Autodesk Inventor part; units mm, degrees
(part 2 of 3)
  line L298 (-57.4722, -60.9676) -> (-57.4397, -60.8956) projected
  line L299 (-57.4397, -60.8956) -> (-57.4038, -60.8255) projected
  line L300 (-57.4038, -60.8255) -> (-57.3646, -60.7575) projected
  line L301 (-57.3646, -60.7575) -> (-57.3224, -60.6916) projected
  line L302 (-57.3224, -60.6916) -> (-57.2771, -60.6279) projected
  line L303 (-57.2771, -60.6279) -> (-57.2288, -60.5665) projected
  line L304 (-57.2288, -60.5665) -> (-57.1777, -60.5075) projected
  line L305 (-57.1777, -60.5075) -> (-57.1239, -60.4511) projected
  line L306 (-57.1239, -60.4511) -> (-57.0675, -60.3973) projected
  line L307 (-57.0675, -60.3973) -> (-57.0085, -60.3462) projected
  line L308 (-57.0085, -60.3462) -> (-56.9471, -60.298) projected
  line L309 (-56.9471, -60.298) -> (-56.8834, -60.2527) projected
  line L310 (-56.8834, -60.2527) -> (-56.8175, -60.2104) projected
  line L311 (-56.8175, -60.2104) -> (-56.7494, -60.1713) projected
  line L312 (-56.7494, -60.1713) -> (-56.6793, -60.1354) projected
  line L313 (-56.6793, -60.1354) -> (-56.6073, -60.1029) projected
  line L314 (-56.6073, -60.1029) -> (-56.5335, -60.0738) projected
  line L315 (-56.5335, -60.0738) -> (-56.458, -60.0483) projected
  line L316 (-56.458, -60.0483) -> (-56.3809, -60.0264) projected
  line L317 (-56.3809, -60.0264) -> (-56.3023, -60.0083) projected
  line L318 (-56.3023, -60.0083) -> (-56.2223, -59.994) projected
  line L319 (-56.2223, -59.994) -> (-56.141, -59.9837) projected
  line L320 (-59.9853, -67.0602) -> (-59.9791, -67.1428) projected
  line L321 (-59.9791, -67.1428) -> (-59.977, -67.2264) projected
  line L322 (-59.977, -67.2264) -> (-59.9792, -67.31) projected
  line L323 (-59.9792, -67.31) -> (-59.9855, -67.3925) projected
  line L324 (-59.9855, -67.3925) -> (-59.9958, -67.4738) projected
  line L325 (-59.9958, -67.4738) -> (-60.0102, -67.5539) projected
  line L326 (-60.0102, -67.5539) -> (-60.0284, -67.6325) projected
  line L327 (-60.0284, -67.6325) -> (-60.0503, -67.7096) projected
  line L328 (-60.0503, -67.7096) -> (-60.0759, -67.7851) projected
  line L329 (-60.0759, -67.7851) -> (-60.105, -67.8588) projected
  line L330 (-60.105, -67.8588) -> (-60.1376, -67.9308) projected
  line L331 (-60.1376, -67.9308) -> (-60.1735, -68.0009) projected
  line L332 (-60.1735, -68.0009) -> (-60.2126, -68.0689) projected
  line L333 (-60.2126, -68.0689) -> (-60.2549, -68.1348) projected
  line L334 (-60.2549, -68.1348) -> (-60.3003, -68.1985) projected
  line L335 (-60.3003, -68.1985) -> (-60.3486, -68.2599) projected
  line L336 (-60.3486, -68.2599) -> (-60.3997, -68.3188) projected
  line L337 (-60.3997, -68.3188) -> (-60.4535, -68.3752) projected
  line L338 (-60.4535, -68.3752) -> (-60.5099, -68.429) projected
  line L339 (-60.5099, -68.429) -> (-60.5689, -68.48) projected
  line L340 (-60.5689, -68.48) -> (-60.6303, -68.5283) projected
  line L341 (-60.6303, -68.5283) -> (-60.6941, -68.5735) projected
  line L342 (-60.6941, -68.5735) -> (-60.76, -68.6158) projected
  line L343 (-60.76, -68.6158) -> (-60.8281, -68.6549) projected
  line L344 (-60.8281, -68.6549) -> (-60.8982, -68.6907) projected
  line L345 (-60.8982, -68.6907) -> (-60.9702, -68.7232) projected
  line L346 (-60.9702, -68.7232) -> (-61.044, -68.7523) projected
  line L347 (-61.044, -68.7523) -> (-61.1195, -68.7778) projected
  line L348 (-61.1195, -68.7778) -> (-61.1966, -68.7997) projected
  line L349 (-61.1966, -68.7997) -> (-61.2752, -68.8178) projected
  line L350 (-61.2752, -68.8178) -> (-61.3553, -68.832) projected
  line L351 (-61.3553, -68.832) -> (-61.4366, -68.8423) projected
  line L352 (-61.4366, -68.8423) -> (-61.5191, -68.8486) projected
  line L353 (-61.5191, -68.8486) -> (-61.6028, -68.8506) projected
  line L354 (-61.6028, -68.8506) -> (-61.6864, -68.8485) projected
  line L355 (-61.6864, -68.8485) -> (-61.7689, -68.8422) projected
  line L356 (-61.7689, -68.8422) -> (-61.8502, -68.8318) projected
  line L357 (-61.8502, -68.8318) -> (-61.9302, -68.8175) projected
  line L358 (-61.9302, -68.8175) -> (-62.0088, -68.7993) projected
  line L359 (-62.0088, -68.7993) -> (-62.0859, -68.7774) projected
  line L360 (-62.0859, -68.7774) -> (-62.1614, -68.7518) projected
  line L361 (-62.1614, -68.7518) -> (-62.2352, -68.7226) projected
  line L362 (-62.2352, -68.7226) -> (-62.3072, -68.6901) projected
  line L363 (-62.3072, -68.6901) -> (-62.3772, -68.6542) projected
  line L364 (-62.3772, -68.6542) -> (-62.4453, -68.615) projected
  line L365 (-62.4453, -68.615) -> (-62.5112, -68.5727) projected
  line L366 (-62.5112, -68.5727) -> (-62.5749, -68.5274) projected
  line L367 (-62.5749, -68.5274) -> (-62.6362, -68.4791) projected
  line L368 (-62.6362, -68.4791) -> (-62.6952, -68.428) projected
  line L369 (-62.6952, -68.428) -> (-62.7516, -68.3742) projected
  line L370 (-62.7516, -68.3742) -> (-62.8054, -68.3177) projected
  line L371 (-62.8054, -68.3177) -> (-62.8564, -68.2587) projected
  line L372 (-62.8564, -68.2587) -> (-62.9046, -68.1973) projected
  line L373 (-62.9046, -68.1973) -> (-62.9499, -68.1336) projected
  line L374 (-62.9499, -68.1336) -> (-62.9921, -68.0676) projected
  line L375 (-62.9921, -68.0676) -> (-63.0312, -67.9996) projected
  line L376 (-63.0312, -67.9996) -> (-63.0671, -67.9295) projected
  line L377 (-63.0671, -67.9295) -> (-63.0996, -67.8575) projected
  line L378 (-63.0996, -67.8575) -> (-63.1287, -67.7837) projected
  line L379 (-63.1287, -67.7837) -> (-63.1542, -67.7082) projected
  line L380 (-63.1542, -67.7082) -> (-63.176, -67.631) projected
  line L381 (-63.176, -67.631) -> (-63.1941, -67.5524) projected
  line L382 (-63.1941, -67.5524) -> (-63.2084, -67.4724) projected
  line L383 (-63.2084, -67.4724) -> (-63.2187, -67.391) projected
  line L384 (-63.2187, -67.391) -> (-63.2249, -67.3085) projected
  line L385 (-63.2249, -67.3085) -> (-63.227, -67.2249) projected
  line L386 (-63.227, -67.2249) -> (-63.2249, -67.1413) projected
  line L387 (-63.2249, -67.1413) -> (-63.2185, -67.0588) projected
  line L388 (-63.2185, -67.0588) -> (-63.2082, -66.9774) projected
  line L389 (-63.2082, -66.9774) -> (-63.1938, -66.8974) projected
  line L390 (-63.1938, -66.8974) -> (-63.1757, -66.8188) projected
  line L391 (-63.1757, -66.8188) -> (-63.1537, -66.7417) projected
  line L392 (-63.1537, -66.7417) -> (-63.1281, -66.6662) projected
  line L393 (-63.1281, -66.6662) -> (-63.099, -66.5924) projected
  line L394 (-63.099, -66.5924) -> (-63.0664, -66.5205) projected
  line L395 (-63.0664, -66.5205) -> (-63.0305, -66.4504) projected
  line L396 (-63.0305, -66.4504) -> (-62.9914, -66.3824) projected
  line L397 (-62.9914, -66.3824) -> (-62.9491, -66.3165) projected
  line L398 (-62.9491, -66.3165) -> (-62.9037, -66.2528) projected
  line L399 (-62.9037, -66.2528) -> (-62.8555, -66.1914) projected
  line L400 (-62.8555, -66.1914) -> (-62.8044, -66.1325) projected
  line L401 (-62.8044, -66.1325) -> (-62.7505, -66.0761) projected
  line L402 (-62.7505, -66.0761) -> (-62.6941, -66.0223) projected
  line L403 (-62.6941, -66.0223) -> (-62.6351, -65.9712) projected
  line L404 (-62.6351, -65.9712) -> (-62.5737, -65.923) projected
  line L405 (-62.5737, -65.923) -> (-62.5099, -65.8777) projected
  line L406 (-62.5099, -65.8777) -> (-62.444, -65.8355) projected
  line L407 (-62.444, -65.8355) -> (-62.3759, -65.7964) projected
  line L408 (-62.3759, -65.7964) -> (-62.3058, -65.7606) projected
  line L409 (-62.3058, -65.7606) -> (-62.2338, -65.7281) projected
  line L410 (-62.2338, -65.7281) -> (-62.16, -65.699) projected
  line L411 (-62.16, -65.699) -> (-62.0845, -65.6735) projected
  line L412 (-62.0845, -65.6735) -> (-62.0074, -65.6516) projected
  line L413 (-62.0074, -65.6516) -> (-61.9288, -65.6335) projected
  line L414 (-61.9288, -65.6335) -> (-61.8487, -65.6193) projected
  line L415 (-61.8487, -65.6193) -> (-61.7674, -65.609) projected
  line L416 (-61.7674, -65.609) -> (-61.6849, -65.6027) projected
  line L417 (-61.6849, -65.6027) -> (-61.6013, -65.6006) projected
  line L418 (-61.6013, -65.6006) -> (-61.5176, -65.6028) projected
  line L419 (-61.5176, -65.6028) -> (-61.4351, -65.6091) projected
  line L420 (-61.4351, -65.6091) -> (-61.3538, -65.6195) projected
  line L421 (-61.3538, -65.6195) -> (-61.2738, -65.6338) projected
  line L422 (-61.2738, -65.6338) -> (-61.1952, -65.652) projected
  line L423 (-61.1952, -65.652) -> (-61.1181, -65.6739) projected
  line L424 (-61.1181, -65.6739) -> (-61.0426, -65.6995) projected
  line L425 (-61.0426, -65.6995) -> (-60.9688, -65.7286) projected
  line L426 (-60.9688, -65.7286) -> (-60.8968, -65.7612) projected
  line L427 (-60.8968, -65.7612) -> (-60.8268, -65.7971) projected
  line L428 (-60.8268, -65.7971) -> (-60.7587, -65.8363) projected
  line L429 (-60.7587, -65.8363) -> (-60.6928, -65.8786) projected
  line L430 (-60.6928, -65.8786) -> (-60.6291, -65.9239) projected
  line L431 (-60.6291, -65.9239) -> (-60.5678, -65.9722) projected
  line L432 (-60.5678, -65.9722) -> (-60.5088, -66.0233) projected
  line L433 (-60.5088, -66.0233) -> (-60.4524, -66.0771) projected
  line L434 (-60.4524, -66.0771) -> (-60.3987, -66.1336) projected
  line L435 (-60.3987, -66.1336) -> (-60.3476, -66.1926) projected
  line L436 (-60.3476, -66.1926) -> (-60.2994, -66.254) projected
  line L437 (-60.2994, -66.254) -> (-60.2541, -66.3177) projected
  line L438 (-60.2541, -66.3177) -> (-60.2119, -66.3837) projected
  line L439 (-60.2119, -66.3837) -> (-60.1728, -66.4517) projected
  line L440 (-60.1728, -66.4517) -> (-60.1369, -66.5218) projected
  line L441 (-60.1369, -66.5218) -> (-60.1044, -66.5938) projected
  line L442 (-60.1044, -66.5938) -> (-60.0754, -66.6676) projected
  line L443 (-60.0754, -66.6676) -> (-60.0498, -66.7431) projected
  line L444 (-60.0498, -66.7431) -> (-60.028, -66.8202) projected
  line L445 (-60.028, -66.8202) -> (-60.0099, -66.8989) projected
  line L446 (-60.0099, -66.8989) -> (-59.9956, -66.9789) projected
  line L447 (-59.9956, -66.9789) -> (-59.9853, -67.0602) projected
  line L448 (-63.2161, -56.1402) -> (-63.2223, -56.0577) projected
  line L449 (-63.2223, -56.0577) -> (-63.2244, -55.9741) projected
  line L450 (-63.2244, -55.9741) -> (-63.2223, -55.8904) projected
  line L451 (-63.2223, -55.8904) -> (-63.216, -55.8079) projected
  line L452 (-63.216, -55.8079) -> (-63.2056, -55.7266) projected
  line L453 (-63.2056, -55.7266) -> (-63.1913, -55.6466) projected
  line L454 (-63.1913, -55.6466) -> (-63.1732, -55.568) projected
  line L455 (-63.1732, -55.568) -> (-63.1512, -55.4909) projected
  line L456 (-63.1512, -55.4909) -> (-63.1257, -55.4154) projected
  line L457 (-63.1257, -55.4154) -> (-63.0966, -55.3416) projected
  line L458 (-63.0966, -55.3416) -> (-63.064, -55.2696) projected
  line L459 (-63.064, -55.2696) -> (-63.0281, -55.1995) projected
  line L460 (-63.0281, -55.1995) -> (-62.9889, -55.1315) projected
  line L461 (-62.9889, -55.1315) -> (-62.9467, -55.0656) projected
  line L462 (-62.9467, -55.0656) -> (-62.9013, -55.0019) projected
  line L463 (-62.9013, -55.0019) -> (-62.8531, -54.9405) projected
  line L464 (-62.8531, -54.9405) -> (-62.802, -54.8816) projected
  line L465 (-62.802, -54.8816) -> (-62.7482, -54.8251) projected
  line L466 (-62.7482, -54.8251) -> (-62.6917, -54.7714) projected
  line L467 (-62.6917, -54.7714) -> (-62.6327, -54.7203) projected
  line L468 (-62.6327, -54.7203) -> (-62.5713, -54.6721) projected
  line L469 (-62.5713, -54.6721) -> (-62.5076, -54.6268) projected
  line L470 (-62.5076, -54.6268) -> (-62.4417, -54.5845) projected
  line L471 (-62.4417, -54.5845) -> (-62.3736, -54.5454) projected
  line L472 (-62.3736, -54.5454) -> (-62.3035, -54.5096) projected
  line L473 (-62.3035, -54.5096) -> (-62.2315, -54.477) projected
  line L474 (-62.2315, -54.477) -> (-62.1577, -54.448) projected
  line L475 (-62.1577, -54.448) -> (-62.0822, -54.4224) projected
  line L476 (-62.0822, -54.4224) -> (-62.0051, -54.4006) projected
  line L477 (-62.0051, -54.4006) -> (-61.9265, -54.3824) projected
  line L478 (-61.9265, -54.3824) -> (-61.8465, -54.3682) projected
  line L479 (-61.8465, -54.3682) -> (-61.7651, -54.3579) projected
  line L480 (-61.7651, -54.3579) -> (-61.6826, -54.3516) projected
  line L481 (-61.6826, -54.3516) -> (-61.599, -54.3495) projected
  line L482 (-61.599, -54.3495) -> (-61.5154, -54.3517) projected
  line L483 (-61.5154, -54.3517) -> (-61.4328, -54.358) projected
  line L484 (-61.4328, -54.358) -> (-61.3515, -54.3683) projected
  line L485 (-61.3515, -54.3683) -> (-61.2715, -54.3826) projected
  line L486 (-61.2715, -54.3826) -> (-61.1929, -54.4008) projected
  line L487 (-61.1929, -54.4008) -> (-61.1158, -54.4227) projected
  line L488 (-61.1158, -54.4227) -> (-61.0403, -54.4483) projected
  line L489 (-61.0403, -54.4483) -> (-60.9665, -54.4774) projected
  line L490 (-60.9665, -54.4774) -> (-60.8945, -54.51) projected
  line L491 (-60.8945, -54.51) -> (-60.8245, -54.5459) projected
  line L492 (-60.8245, -54.5459) -> (-60.7564, -54.585) projected
  line L493 (-60.7564, -54.585) -> (-60.6905, -54.6273) projected
  line L494 (-60.6905, -54.6273) -> (-60.6268, -54.6726) projected
  line L495 (-60.6268, -54.6726) -> (-60.5654, -54.7209) projected
  line L496 (-60.5654, -54.7209) -> (-60.5065, -54.772) projected
  line L497 (-60.5065, -54.772) -> (-60.4501, -54.8258) projected
  line L498 (-60.4501, -54.8258) -> (-60.3963, -54.8822) projected
  line L499 (-60.3963, -54.8822) -> (-60.3452, -54.9412) projected
  line L500 (-60.3452, -54.9412) -> (-60.297, -55.0026) projected
  line L501 (-60.297, -55.0026) -> (-60.2517, -55.0663) projected
  line L502 (-60.2517, -55.0663) -> (-60.2095, -55.1323) projected
  line L503 (-60.2095, -55.1323) -> (-60.1703, -55.2003) projected
  line L504 (-60.1703, -55.2003) -> (-60.1345, -55.2704) projected
  line L505 (-60.1345, -55.2704) -> (-60.102, -55.3424) projected
  line L506 (-60.102, -55.3424) -> (-60.0729, -55.4162) projected
  line L507 (-60.0729, -55.4162) -> (-60.0474, -55.4917) projected
  line L508 (-60.0474, -55.4917) -> (-60.0255, -55.5688) projected
  line L509 (-60.0255, -55.5688) -> (-60.0074, -55.6475) projected
  line L510 (-60.0074, -55.6475) -> (-59.9931, -55.7275) projected
  line L511 (-59.9931, -55.7275) -> (-59.9828, -55.8088) projected
  line L512 (-59.9828, -55.8088) -> (-59.9765, -55.8914) projected
  line L513 (-59.9765, -55.8914) -> (-59.9744, -55.975) projected
  line L514 (-59.9744, -55.975) -> (-59.9766, -56.0586) projected
  line L515 (-59.9766, -56.0586) -> (-59.9829, -56.1411) projected
  line L516 (-59.9829, -56.1411) -> (-59.9932, -56.2224) projected
  line L517 (-59.9932, -56.2224) -> (-60.0075, -56.3025) projected
  line L518 (-60.0075, -56.3025) -> (-60.0257, -56.3811) projected
  line L519 (-60.0257, -56.3811) -> (-60.0476, -56.4582) projected
  line L520 (-60.0476, -56.4582) -> (-60.0732, -56.5337) projected
  line L521 (-60.0732, -56.5337) -> (-60.1023, -56.6075) projected
  line L522 (-60.1023, -56.6075) -> (-60.1349, -56.6794) projected
  line L523 (-60.1349, -56.6794) -> (-60.1708, -56.7495) projected
  line L524 (-60.1708, -56.7495) -> (-60.2099, -56.8175) projected
  line L525 (-60.2099, -56.8175) -> (-60.2522, -56.8834) projected
  line L526 (-60.2522, -56.8834) -> (-60.2975, -56.9471) projected
  line L527 (-60.2975, -56.9471) -> (-60.3458, -57.0085) projected
  line L528 (-60.3458, -57.0085) -> (-60.3969, -57.0675) projected
  line L529 (-60.3969, -57.0675) -> (-60.4507, -57.1239) projected
  line L530 (-60.4507, -57.1239) -> (-60.5072, -57.1777) projected
  line L531 (-60.5072, -57.1777) -> (-60.5661, -57.2287) projected
  line L532 (-60.5661, -57.2287) -> (-60.6275, -57.277) projected
  line L533 (-60.6275, -57.277) -> (-60.6913, -57.3222) projected
  line L534 (-60.6913, -57.3222) -> (-60.7572, -57.3645) projected
  line L535 (-60.7572, -57.3645) -> (-60.8253, -57.4036) projected
  line L536 (-60.8253, -57.4036) -> (-60.8953, -57.4395) projected
  line L537 (-60.8953, -57.4395) -> (-60.9673, -57.472) projected
  line L538 (-60.9673, -57.472) -> (-61.0411, -57.5011) projected
  line L539 (-61.0411, -57.5011) -> (-61.1166, -57.5266) projected
  line L540 (-61.1166, -57.5266) -> (-61.1938, -57.5485) projected
  line L541 (-61.1938, -57.5485) -> (-61.2724, -57.5666) projected
  line L542 (-61.2724, -57.5666) -> (-61.3524, -57.5809) projected
  line L543 (-61.3524, -57.5809) -> (-61.4337, -57.5912) projected
  line L544 (-61.4337, -57.5912) -> (-61.5163, -57.5974) projected
  line L545 (-61.5163, -57.5974) -> (-61.5999, -57.5995) projected
  line L546 (-61.5999, -57.5995) -> (-61.6835, -57.5974) projected
  line L547 (-61.6835, -57.5974) -> (-61.766, -57.5911) projected
  line L548 (-61.766, -57.5911) -> (-61.8474, -57.5807) projected
  line L549 (-61.8474, -57.5807) -> (-61.9274, -57.5664) projected
  line L550 (-61.9274, -57.5664) -> (-62.006, -57.5482) projected
  line L551 (-62.006, -57.5482) -> (-62.0831, -57.5263) projected
  line L552 (-62.0831, -57.5263) -> (-62.1586, -57.5008) projected
  line L553 (-62.1586, -57.5008) -> (-62.2324, -57.4716) projected
  line L554 (-62.2324, -57.4716) -> (-62.3044, -57.4391) projected
  line L555 (-62.3044, -57.4391) -> (-62.3744, -57.4032) projected
  line L556 (-62.3744, -57.4032) -> (-62.4424, -57.364) projected
  line L557 (-62.4424, -57.364) -> (-62.5084, -57.3217) projected
  line L558 (-62.5084, -57.3217) -> (-62.5721, -57.2764) projected
  line L559 (-62.5721, -57.2764) -> (-62.6334, -57.2282) projected
  line L560 (-62.6334, -57.2282) -> (-62.6924, -57.1771) projected
  line L561 (-62.6924, -57.1771) -> (-62.7488, -57.1232) projected
  line L562 (-62.7488, -57.1232) -> (-62.8026, -57.0668) projected
  line L563 (-62.8026, -57.0668) -> (-62.8537, -57.0078) projected
  line L564 (-62.8537, -57.0078) -> (-62.9019, -56.9464) projected
  line L565 (-62.9019, -56.9464) -> (-62.9472, -56.8827) projected
  line L566 (-62.9472, -56.8827) -> (-62.9894, -56.8167) projected
  line L567 (-62.9894, -56.8167) -> (-63.0285, -56.7487) projected
  line L568 (-63.0285, -56.7487) -> (-63.0644, -56.6786) projected
  line L569 (-63.0644, -56.6786) -> (-63.0969, -56.6066) projected
  line L570 (-63.0969, -56.6066) -> (-63.126, -56.5328) projected
  line L571 (-63.126, -56.5328) -> (-63.1515, -56.4573) projected
  line L572 (-63.1515, -56.4573) -> (-63.1734, -56.3802) projected
  line L573 (-63.1734, -56.3802) -> (-63.1915, -56.3016) projected
  line L574 (-63.1915, -56.3016) -> (-63.2058, -56.2215) projected
  line L575 (-63.2058, -56.2215) -> (-63.2161, -56.1402) projected
  arc A0 (-52.9038, -71.2653) -> (-48.6, -61.6029) centre (-61.5843, -61.6091) ccw projected
  arc A1 (-48.6, -61.6029) -> (-48.8055, -59.2842) centre (-61.5557, -61.583) ccw projected
  arc A2 (-48.8055, -59.2842) -> (-59.1805, -48.8249) centre (-61.5989, -61.5991) ccw projected
  arc A3 (-59.1805, -48.8249) -> (-74.163, -58.2471) centre (-61.5986, -61.6031) ccw projected
  arc A4 (-74.163, -58.2471) -> (-72.8082, -68.1903) centre (-61.5989, -61.5991) ccw projected
  arc A5 (-72.8082, -68.1903) -> (-52.9038, -71.2653) centre (-61.6004, -61.5999) ccw projected
  point P0 (0, 0)
ref_plane "Work Plane1" through (0, 0, 0) normal (0, 0, 1) x (1, 0, 0)
sketch "Sketch5" plane through (0, 0, 0) normal (0, 0, 1) x (1, 0, 0)
  line L0 (67.06, -63.215) -> (67.1425, -63.2212) projected
  line L1 (67.1425, -63.2212) -> (67.2261, -63.2233) projected
  line L2 (67.2261, -63.2233) -> (67.3097, -63.2211) projected
  line L3 (67.3097, -63.2211) -> (67.3923, -63.2148) projected
  line L4 (67.3923, -63.2148) -> (67.4736, -63.2045) projected
  line L5 (67.4736, -63.2045) -> (67.5536, -63.1902) projected
  line L6 (67.5536, -63.1902) -> (67.6322, -63.172) projected
  line L7 (67.6322, -63.172) -> (67.7093, -63.15) projected
  line L8 (67.7093, -63.15) -> (67.7848, -63.1245) projected
  line L9 (67.7848, -63.1245) -> (67.8586, -63.0953) projected
  line L10 (67.8586, -63.0953) -> (67.9306, -63.0628) projected
  line L11 (67.9306, -63.0628) -> (68.0006, -63.0269) projected
  line L12 (68.0006, -63.0269) -> (68.0686, -62.9877) projected
  line L13 (68.0686, -62.9877) -> (68.1346, -62.9454) projected
  line L14 (68.1346, -62.9454) -> (68.1982, -62.9001) projected
  line L15 (68.1982, -62.9001) -> (68.2596, -62.8518) projected
  line L16 (68.2596, -62.8518) -> (68.3186, -62.8007) projected
  line L17 (68.3186, -62.8007) -> (68.375, -62.7469) projected
  line L18 (68.375, -62.7469) -> (68.4288, -62.6904) projected
  line L19 (68.4288, -62.6904) -> (68.4798, -62.6314) projected
  line L20 (68.4798, -62.6314) -> (68.528, -62.57) projected
  line L21 (68.528, -62.57) -> (68.5733, -62.5063) projected
  line L22 (68.5733, -62.5063) -> (68.6155, -62.4404) projected
  line L23 (68.6155, -62.4404) -> (68.6546, -62.3723) projected
  line L24 (68.6546, -62.3723) -> (68.6905, -62.3022) projected
  line L25 (68.6905, -62.3022) -> (68.723, -62.2302) projected
  line L26 (68.723, -62.2302) -> (68.7521, -62.1564) projected
  line L27 (68.7521, -62.1564) -> (68.7776, -62.0809) projected
  line L28 (68.7776, -62.0809) -> (68.7995, -62.0038) projected
  line L29 (68.7995, -62.0038) -> (68.8176, -61.9252) projected
  line L30 (68.8176, -61.9252) -> (68.8318, -61.8451) projected
  line L31 (68.8318, -61.8451) -> (68.8421, -61.7638) projected
  line L32 (68.8421, -61.7638) -> (68.8484, -61.6813) projected
  line L33 (68.8484, -61.6813) -> (68.8505, -61.5976) projected
  line L34 (68.8505, -61.5976) -> (68.8483, -61.514) projected
  line L35 (68.8483, -61.514) -> (68.842, -61.4315) projected
  line L36 (68.842, -61.4315) -> (68.8316, -61.3502) projected
  line L37 (68.8316, -61.3502) -> (68.8173, -61.2702) projected
  line L38 (68.8173, -61.2702) -> (68.7991, -61.1916) projected
  line L39 (68.7991, -61.1916) -> (68.7772, -61.1144) projected
  line L40 (68.7772, -61.1144) -> (68.7516, -61.039) projected
  line L41 (68.7516, -61.039) -> (68.7225, -60.9652) projected
  line L42 (68.7225, -60.9652) -> (68.6899, -60.8932) projected
  line L43 (68.6899, -60.8932) -> (68.654, -60.8232) projected
  line L44 (68.654, -60.8232) -> (68.6149, -60.7551) projected
  line L45 (68.6149, -60.7551) -> (68.5726, -60.6892) projected
  line L46 (68.5726, -60.6892) -> (68.5272, -60.6255) projected
  line L47 (68.5272, -60.6255) -> (68.479, -60.5641) projected
  line L48 (68.479, -60.5641) -> (68.4279, -60.5052) projected
  line L49 (68.4279, -60.5052) -> (68.374, -60.4488) projected
  line L50 (68.374, -60.4488) -> (68.3176, -60.395) projected
  line L51 (68.3176, -60.395) -> (68.2586, -60.344) projected
  line L52 (68.2586, -60.344) -> (68.1972, -60.2957) projected
  line L53 (68.1972, -60.2957) -> (68.1335, -60.2505) projected
  line L54 (68.1335, -60.2505) -> (68.0675, -60.2082) projected
  line L55 (68.0675, -60.2082) -> (67.9995, -60.1691) projected
  line L56 (67.9995, -60.1691) -> (67.9294, -60.1333) projected
  line L57 (67.9294, -60.1333) -> (67.8574, -60.1007) projected
  line L58 (67.8574, -60.1007) -> (67.7836, -60.0717) projected
  line L59 (67.7836, -60.0717) -> (67.7081, -60.0462) projected
  line L60 (67.7081, -60.0462) -> (67.6309, -60.0243) projected
  line L61 (67.6309, -60.0243) -> (67.5523, -60.0062) projected
  line L62 (67.5523, -60.0062) -> (67.4723, -59.9919) projected
  line L63 (67.4723, -59.9919) -> (67.391, -59.9816) projected
  line L64 (67.391, -59.9816) -> (67.3084, -59.9754) projected
  line L65 (67.3084, -59.9754) -> (67.2248, -59.9733) projected
  line L66 (67.2248, -59.9733) -> (67.1412, -59.9754) projected
  line L67 (67.1412, -59.9754) -> (67.0587, -59.9818) projected
  line L68 (67.0587, -59.9818) -> (66.9773, -59.9921) projected
  line L69 (66.9773, -59.9921) -> (66.8973, -60.0064) projected
  line L70 (66.8973, -60.0064) -> (66.8187, -60.0246) projected
  line L71 (66.8187, -60.0246) -> (66.7416, -60.0465) projected
  line L72 (66.7416, -60.0465) -> (66.6661, -60.0721) projected
  line L73 (66.6661, -60.0721) -> (66.5923, -60.1013) projected
  line L74 (66.5923, -60.1013) -> (66.5204, -60.1338) projected
  line L75 (66.5204, -60.1338) -> (66.4503, -60.1697) projected
  line L76 (66.4503, -60.1697) -> (66.3823, -60.2089) projected
  line L77 (66.3823, -60.2089) -> (66.3164, -60.2512) projected
  line L78 (66.3164, -60.2512) -> (66.2527, -60.2965) projected
  line L79 (66.2527, -60.2965) -> (66.1913, -60.3448) projected
  line L80 (66.1913, -60.3448) -> (66.1324, -60.3959) projected
  line L81 (66.1324, -60.3959) -> (66.0759, -60.4497) projected
  line L82 (66.0759, -60.4497) -> (66.0222, -60.5062) projected
  line L83 (66.0222, -60.5062) -> (65.9711, -60.5652) projected
  line L84 (65.9711, -60.5652) -> (65.9229, -60.6266) projected
  line L85 (65.9229, -60.6266) -> (65.8776, -60.6903) projected
  line L86 (65.8776, -60.6903) -> (65.8354, -60.7562) projected
  line L87 (65.8354, -60.7562) -> (65.7963, -60.8243) projected
  line L88 (65.7963, -60.8243) -> (65.7604, -60.8944) projected
  line L89 (65.7604, -60.8944) -> (65.7279, -60.9664) projected
  line L90 (65.7279, -60.9664) -> (65.6988, -61.0402) projected
  line L91 (65.6988, -61.0402) -> (65.6733, -61.1157) projected
  line L92 (65.6733, -61.1157) -> (65.6515, -61.1928) projected
  line L93 (65.6515, -61.1928) -> (65.6333, -61.2714) projected
  line L94 (65.6333, -61.2714) -> (65.6191, -61.3515) projected
  line L95 (65.6191, -61.3515) -> (65.6088, -61.4328) projected
  line L96 (65.6088, -61.4328) -> (65.6025, -61.5153) projected
  line L97 (65.6025, -61.5153) -> (65.6005, -61.599) projected
  line L98 (65.6005, -61.599) -> (65.6026, -61.6826) projected
  line L99 (65.6026, -61.6826) -> (65.6089, -61.7651) projected
  line L100 (65.6089, -61.7651) -> (65.6193, -61.8464) projected
  line L101 (65.6193, -61.8464) -> (65.6336, -61.9264) projected
  line L102 (65.6336, -61.9264) -> (65.6518, -62.005) projected
  line L103 (65.6518, -62.005) -> (65.6737, -62.0821) projected
  line L104 (65.6737, -62.0821) -> (65.6993, -62.1576) projected
  line L105 (65.6993, -62.1576) -> (65.7284, -62.2314) projected
  line L106 (65.7284, -62.2314) -> (65.761, -62.3034) projected
  line L107 (65.761, -62.3034) -> (65.7969, -62.3734) projected
  line L108 (65.7969, -62.3734) -> (65.8361, -62.4415) projected
  line L109 (65.8361, -62.4415) -> (65.8783, -62.5074) projected
  line L110 (65.8783, -62.5074) -> (65.9237, -62.5711) projected
  line L111 (65.9237, -62.5711) -> (65.9719, -62.6325) projected
  line L112 (65.9719, -62.6325) -> (66.023, -62.6914) projected
  line L113 (66.023, -62.6914) -> (66.0769, -62.7478) projected
  line L114 (66.0769, -62.7478) -> (66.1333, -62.8016) projected
  line L115 (66.1333, -62.8016) -> (66.1923, -62.8526) projected
  line L116 (66.1923, -62.8526) -> (66.2537, -62.9009) projected
  line L117 (66.2537, -62.9009) -> (66.3174, -62.9461) projected
  line L118 (66.3174, -62.9461) -> (66.3834, -62.9884) projected
  line L119 (66.3834, -62.9884) -> (66.4515, -63.0275) projected
  line L120 (66.4515, -63.0275) -> (66.5215, -63.0633) projected
  line L121 (66.5215, -63.0633) -> (66.5935, -63.0959) projected
  line L122 (66.5935, -63.0959) -> (66.6673, -63.1249) projected
  line L123 (66.6673, -63.1249) -> (66.7429, -63.1504) projected
  line L124 (66.7429, -63.1504) -> (66.82, -63.1723) projected
  line L125 (66.82, -63.1723) -> (66.8986, -63.1904) projected
  line L126 (66.8986, -63.1904) -> (66.9786, -63.2047) projected
  line L127 (66.9786, -63.2047) -> (67.06, -63.215) projected
  line L128 (56.141, -59.9837) -> (56.0584, -59.9774) projected
  line L129 (56.0584, -59.9774) -> (55.9748, -59.9753) projected
  line L130 (55.9748, -59.9753) -> (55.8912, -59.9774) projected
  line L131 (55.8912, -59.9774) -> (55.8087, -59.9837) projected
  line L132 (55.8087, -59.9837) -> (55.7273, -59.994) projected
  line L133 (55.7273, -59.994) -> (55.6473, -60.0083) projected
  line L134 (55.6473, -60.0083) -> (55.5687, -60.0265) projected
  line L135 (55.5687, -60.0265) -> (55.4916, -60.0484) projected
  line L136 (55.4916, -60.0484) -> (55.4161, -60.074) projected
  line L137 (55.4161, -60.074) -> (55.3423, -60.1031) projected
  line L138 (55.3423, -60.1031) -> (55.2703, -60.1356) projected
  line L139 (55.2703, -60.1356) -> (55.2003, -60.1715) projected
  line L140 (55.2003, -60.1715) -> (55.1322, -60.2106) projected
  line L141 (55.1322, -60.2106) -> (55.0663, -60.2529) projected
  line L142 (55.0663, -60.2529) -> (55.0026, -60.2982) projected
  line L143 (55.0026, -60.2982) -> (54.9412, -60.3465) projected
  line L144 (54.9412, -60.3465) -> (54.8822, -60.3976) projected
  line L145 (54.8822, -60.3976) -> (54.8258, -60.4514) projected
  line L146 (54.8258, -60.4514) -> (54.772, -60.5078) projected
  line L147 (54.772, -60.5078) -> (54.7209, -60.5668) projected
  line L148 (54.7209, -60.5668) -> (54.6727, -60.6282) projected
  line L149 (54.6727, -60.6282) -> (54.6274, -60.6919) projected
  line L150 (54.6274, -60.6919) -> (54.5852, -60.7578) projected
  line L151 (54.5852, -60.7578) -> (54.546, -60.8259) projected
  line L152 (54.546, -60.8259) -> (54.5102, -60.8959) projected
  line L153 (54.5102, -60.8959) -> (54.4776, -60.9679) projected
  line L154 (54.4776, -60.9679) -> (54.4485, -61.0417) projected
  line L155 (54.4485, -61.0417) -> (54.423, -61.1172) projected
  line L156 (54.423, -61.1172) -> (54.4011, -61.1944) projected
  line L157 (54.4011, -61.1944) -> (54.383, -61.273) projected
  line L158 (54.383, -61.273) -> (54.3687, -61.353) projected
  line L159 (54.3687, -61.353) -> (54.3584, -61.4343) projected
  line L160 (54.3584, -61.4343) -> (54.3521, -61.5169) projected
  line L161 (54.3521, -61.5169) -> (54.35, -61.6005) projected
  line L162 (54.35, -61.6005) -> (54.3521, -61.6841) projected
  line L163 (54.3521, -61.6841) -> (54.3584, -61.7666) projected
  line L164 (54.3584, -61.7666) -> (54.3688, -61.8479) projected
  line L165 (54.3688, -61.8479) -> (54.3831, -61.928) projected
  line L166 (54.3831, -61.928) -> (54.4012, -62.0066) projected
  line L167 (54.4012, -62.0066) -> (54.4231, -62.0837) projected
  line L168 (54.4231, -62.0837) -> (54.4487, -62.1592) projected
  line L169 (54.4487, -62.1592) -> (54.4778, -62.233) projected
  line L170 (54.4778, -62.233) -> (54.5103, -62.305) projected
  line L171 (54.5103, -62.305) -> (54.5462, -62.375) projected
  line L172 (54.5462, -62.375) -> (54.5854, -62.4431) projected
  line L173 (54.5854, -62.4431) -> (54.6276, -62.509) projected
  line L174 (54.6276, -62.509) -> (54.6729, -62.5727) projected
  line L175 (54.6729, -62.5727) -> (54.7212, -62.6341) projected
  line L176 (54.7212, -62.6341) -> (54.7723, -62.693) projected
  line L177 (54.7723, -62.693) -> (54.8261, -62.7495) projected
  line L178 (54.8261, -62.7495) -> (54.8825, -62.8033) projected
  line L179 (54.8825, -62.8033) -> (54.9415, -62.8543) projected
  line L180 (54.9415, -62.8543) -> (55.0029, -62.9026) projected
  line L181 (55.0029, -62.9026) -> (55.0666, -62.9479) projected
  line L182 (55.0666, -62.9479) -> (55.1325, -62.9901) projected
  line L183 (55.1325, -62.9901) -> (55.2006, -63.0292) projected
  line L184 (55.2006, -63.0292) -> (55.2707, -63.0651) projected
  line L185 (55.2707, -63.0651) -> (55.3427, -63.0977) projected
  line L186 (55.3427, -63.0977) -> (55.4165, -63.1267) projected
  line L187 (55.4165, -63.1267) -> (55.492, -63.1523) projected
  line L188 (55.492, -63.1523) -> (55.5691, -63.1742) projected
  line L189 (55.5691, -63.1742) -> (55.6477, -63.1923) projected
  line L190 (55.6477, -63.1923) -> (55.7277, -63.2066) projected
  line L191 (55.7277, -63.2066) -> (55.809, -63.2169) projected
  line L192 (55.809, -63.2169) -> (55.8916, -63.2232) projected
  line L193 (55.8916, -63.2232) -> (55.9752, -63.2253) projected
  line L194 (55.9752, -63.2253) -> (56.0588, -63.2232) projected
  line L195 (56.0588, -63.2232) -> (56.1413, -63.2169) projected
  line L196 (56.1413, -63.2169) -> (56.2227, -63.2065) projected
  line L197 (56.2227, -63.2065) -> (56.3027, -63.1922) projected
  line L198 (56.3027, -63.1922) -> (56.3813, -63.1741) projected
  line L199 (56.3813, -63.1741) -> (56.4584, -63.1522) projected
  line L200 (56.4584, -63.1522) -> (56.5339, -63.1266) projected
  line L201 (56.5339, -63.1266) -> (56.6077, -63.0975) projected
  line L202 (56.6077, -63.0975) -> (56.6797, -63.065) projected
  line L203 (56.6797, -63.065) -> (56.7497, -63.0291) projected
  line L204 (56.7497, -63.0291) -> (56.8178, -62.9899) projected
  line L205 (56.8178, -62.9899) -> (56.8837, -62.9476) projected
  line L206 (56.8837, -62.9476) -> (56.9474, -62.9023) projected
  line L207 (56.9474, -62.9023) -> (57.0088, -62.8541) projected
  line L208 (57.0088, -62.8541) -> (57.0678, -62.803) projected
  line L209 (57.0678, -62.803) -> (57.1242, -62.7492) projected
  line L210 (57.1242, -62.7492) -> (57.178, -62.6928) projected
  line L211 (57.178, -62.6928) -> (57.2291, -62.6338) projected
  line L212 (57.2291, -62.6338) -> (57.2773, -62.5724) projected
  line L213 (57.2773, -62.5724) -> (57.3226, -62.5087) projected
  line L214 (57.3226, -62.5087) -> (57.3648, -62.4427) projected
  line L215 (57.3648, -62.4427) -> (57.404, -62.3747) projected
  line L216 (57.404, -62.3747) -> (57.4398, -62.3046) projected
  line L217 (57.4398, -62.3046) -> (57.4724, -62.2326) projected
  line L218 (57.4724, -62.2326) -> (57.5015, -62.1588) projected
  line L219 (57.5015, -62.1588) -> (57.527, -62.0833) projected
  line L220 (57.527, -62.0833) -> (57.5489, -62.0062) projected
  line L221 (57.5489, -62.0062) -> (57.567, -61.9276) projected
  line L222 (57.567, -61.9276) -> (57.5813, -61.8476) projected
  line L223 (57.5813, -61.8476) -> (57.5916, -61.7662) projected
  line L224 (57.5916, -61.7662) -> (57.5979, -61.6837) projected
  line L225 (57.5979, -61.6837) -> (57.6, -61.6001) projected
  line L226 (57.6, -61.6001) -> (57.5979, -61.5165) projected
  line L227 (57.5979, -61.5165) -> (57.5916, -61.4339) projected
  line L228 (57.5916, -61.4339) -> (57.5812, -61.3526) projected
  line L229 (57.5812, -61.3526) -> (57.5669, -61.2726) projected
  line L230 (57.5669, -61.2726) -> (57.5488, -61.194) projected
  line L231 (57.5488, -61.194) -> (57.5269, -61.1169) projected
  line L232 (57.5269, -61.1169) -> (57.5013, -61.0414) projected
  line L233 (57.5013, -61.0414) -> (57.4722, -60.9676) projected
  line L234 (57.4722, -60.9676) -> (57.4397, -60.8956) projected
  line L235 (57.4397, -60.8956) -> (57.4038, -60.8255) projected
  line L236 (57.4038, -60.8255) -> (57.3646, -60.7575) projected
  line L237 (57.3646, -60.7575) -> (57.3224, -60.6916) projected
  line L238 (57.3224, -60.6916) -> (57.2771, -60.6279) projected
  line L239 (57.2771, -60.6279) -> (57.2288, -60.5665) projected
  line L240 (57.2288, -60.5665) -> (57.1777, -60.5075) projected
  line L241 (57.1777, -60.5075) -> (57.1239, -60.4511) projected
  line L242 (57.1239, -60.4511) -> (57.0675, -60.3973) projected
  line L243 (57.0675, -60.3973) -> (57.0085, -60.3462) projected
  line L244 (57.0085, -60.3462) -> (56.9471, -60.298) projected
  line L245 (56.9471, -60.298) -> (56.8834, -60.2527) projected
  line L246 (56.8834, -60.2527) -> (56.8175, -60.2104) projected
  line L247 (56.8175, -60.2104) -> (56.7494, -60.1713) projected
  line L248 (56.7494, -60.1713) -> (56.6793, -60.1354) projected
  line L249 (56.6793, -60.1354) -> (56.6073, -60.1029) projected
  line L250 (56.6073, -60.1029) -> (56.5335, -60.0738) projected
  line L251 (56.5335, -60.0738) -> (56.458, -60.0483) projected
  line L252 (56.458, -60.0483) -> (56.3809, -60.0264) projected
  line L253 (56.3809, -60.0264) -> (56.3023, -60.0083) projected
  line L254 (56.3023, -60.0083) -> (56.2223, -59.994) projected
  line L255 (56.2223, -59.994) -> (56.141, -59.9837) projected
  line L256 (63.2161, -56.1402) -> (63.2223, -56.0577) projected
  line L257 (63.2223, -56.0577) -> (63.2244, -55.9741) projected
  line L258 (63.2244, -55.9741) -> (63.2223, -55.8904) projected
  line L259 (63.2223, -55.8904) -> (63.216, -55.8079) projected
  line L260 (63.216, -55.8079) -> (63.2056, -55.7266) projected
  line L261 (63.2056, -55.7266) -> (63.1913, -55.6466) projected
  line L262 (63.1913, -55.6466) -> (63.1732, -55.568) projected
  line L263 (63.1732, -55.568) -> (63.1512, -55.4909) projected
  line L264 (63.1512, -55.4909) -> (63.1257, -55.4154) projected
  line L265 (63.1257, -55.4154) -> (63.0966, -55.3416) projected
  line L266 (63.0966, -55.3416) -> (63.064, -55.2696) projected
  line L267 (63.064, -55.2696) -> (63.0281, -55.1995) projected
  line L268 (63.0281, -55.1995) -> (62.9889, -55.1315) projected
  line L269 (62.9889, -55.1315) -> (62.9467, -55.0656) projected
  line L270 (62.9467, -55.0656) -> (62.9013, -55.0019) projected
  line L271 (62.9013, -55.0019) -> (62.8531, -54.9405) projected
  line L272 (62.8531, -54.9405) -> (62.802, -54.8816) projected
  line L273 (62.802, -54.8816) -> (62.7482, -54.8251) projected
  line L274 (62.7482, -54.8251) -> (62.6917, -54.7714) projected
  line L275 (62.6917, -54.7714) -> (62.6327, -54.7203) projected
  line L276 (62.6327, -54.7203) -> (62.5713, -54.6721) projected
  line L277 (62.5713, -54.6721) -> (62.5076, -54.6268) projected
  line L278 (62.5076, -54.6268) -> (62.4417, -54.5845) projected
  line L279 (62.4417, -54.5845) -> (62.3736, -54.5454) projected
  line L280 (62.3736, -54.5454) -> (62.3035, -54.5096) projected
  line L281 (62.3035, -54.5096) -> (62.2315, -54.477) projected
  line L282 (62.2315, -54.477) -> (62.1577, -54.448) projected
  line L283 (62.1577, -54.448) -> (62.0822, -54.4224) projected
  line L284 (62.0822, -54.4224) -> (62.0051, -54.4006) projected
  line L285 (62.0051, -54.4006) -> (61.9265, -54.3824) projected
  line L286 (61.9265, -54.3824) -> (61.8465, -54.3682) projected
  line L287 (61.8465, -54.3682) -> (61.7651, -54.3579) projected
  line L288 (61.7651, -54.3579) -> (61.6826, -54.3516) projected
  line L289 (61.6826, -54.3516) -> (61.599, -54.3495) projected
  line L290 (61.599, -54.3495) -> (61.5154, -54.3517) projected
  line L291 (61.5154, -54.3517) -> (61.4328, -54.358) projected
  line L292 (61.4328, -54.358) -> (61.3515, -54.3683) projected
  line L293 (61.3515, -54.3683) -> (61.2715, -54.3826) projected
  line L294 (61.2715, -54.3826) -> (61.1929, -54.4008) projected
  line L295 (61.1929, -54.4008) -> (61.1158, -54.4227) projected
  line L296 (61.1158, -54.4227) -> (61.0403, -54.4483) projected
  line L297 (61.0403, -54.4483) -> (60.9665, -54.4774) projected
  line L298 (60.9665, -54.4774) -> (60.8945, -54.51) projected
  line L299 (60.8945, -54.51) -> (60.8245, -54.5459) projected
  line L300 (60.8245, -54.5459) -> (60.7564, -54.585) projected
  line L301 (60.7564, -54.585) -> (60.6905, -54.6273) projected
  line L302 (60.6905, -54.6273) -> (60.6268, -54.6726) projected
  line L303 (60.6268, -54.6726) -> (60.5654, -54.7209) projected
  line L304 (60.5654, -54.7209) -> (60.5065, -54.772) projected
  line L305 (60.5065, -54.772) -> (60.4501, -54.8258) projected
  line L306 (60.4501, -54.8258) -> (60.3963, -54.8822) projected
  line L307 (60.3963, -54.8822) -> (60.3452, -54.9412) projected
  line L308 (60.3452, -54.9412) -> (60.297, -55.0026) projected
  line L309 (60.297, -55.0026) -> (60.2517, -55.0663) projected
  line L310 (60.2517, -55.0663) -> (60.2095, -55.1323) projected
  line L311 (60.2095, -55.1323) -> (60.1703, -55.2003) projected
  line L312 (60.1703, -55.2003) -> (60.1345, -55.2704) projected
  line L313 (60.1345, -55.2704) -> (60.102, -55.3424) projected
  line L314 (60.102, -55.3424) -> (60.0729, -55.4162) projected
  line L315 (60.0729, -55.4162) -> (60.0474, -55.4917) projected
  line L316 (60.0474, -55.4917) -> (60.0255, -55.5688) projected
  line L317 (60.0255, -55.5688) -> (60.0074, -55.6475) projected
  line L318 (60.0074, -55.6475) -> (59.9931, -55.7275) projected
  line L319 (59.9931, -55.7275) -> (59.9828, -55.8088) projected
  line L320 (59.9828, -55.8088) -> (59.9765, -55.8914) projected
  line L321 (59.9765, -55.8914) -> (59.9744, -55.975) projected
  line L322 (59.9744, -55.975) -> (59.9766, -56.0586) projected
  line L323 (59.9766, -56.0586) -> (59.9829, -56.1411) projected
  line L324 (59.9829, -56.1411) -> (59.9932, -56.2224) projected
  line L325 (59.9932, -56.2224) -> (60.0075, -56.3025) projected
  line L326 (60.0075, -56.3025) -> (60.0257, -56.3811) projected
  line L327 (60.0257, -56.3811) -> (60.0476, -56.4582) projected
  line L328 (60.0476, -56.4582) -> (60.0732, -56.5337) projected
  line L329 (60.0732, -56.5337) -> (60.1023, -56.6075) projected
  line L330 (60.1023, -56.6075) -> (60.1349, -56.6794) projected
  line L331 (60.1349, -56.6794) -> (60.1708, -56.7495) projected
  line L332 (60.1708, -56.7495) -> (60.2099, -56.8175) projected
  line L333 (60.2099, -56.8175) -> (60.2522, -56.8834) projected
  line L334 (60.2522, -56.8834) -> (60.2975, -56.9471) projected
  line L335 (60.2975, -56.9471) -> (60.3458, -57.0085) projected
  line L336 (60.3458, -57.0085) -> (60.3969, -57.0675) projected
  line L337 (60.3969, -57.0675) -> (60.4507, -57.1239) projected
  line L338 (60.4507, -57.1239) -> (60.5072, -57.1777) projected
  line L339 (60.5072, -57.1777) -> (60.5661, -57.2287) projected
  line L340 (60.5661, -57.2287) -> (60.6275, -57.277) projected
  line L341 (60.6275, -57.277) -> (60.6913, -57.3222) projected
  line L342 (60.6913, -57.3222) -> (60.7572, -57.3645) projected
  line L343 (60.7572, -57.3645) -> (60.8253, -57.4036) projected
  line L344 (60.8253, -57.4036) -> (60.8953, -57.4395) projected
  line L345 (60.8953, -57.4395) -> (60.9673, -57.472) projected
  line L346 (60.9673, -57.472) -> (61.0411, -57.5011) projected
  line L347 (61.0411, -57.5011) -> (61.1166, -57.5266) projected
  line L348 (61.1166, -57.5266) -> (61.1938, -57.5485) projected
  line L349 (61.1938, -57.5485) -> (61.2724, -57.5666) projected
  line L350 (61.2724, -57.5666) -> (61.3524, -57.5809) projected
  line L351 (61.3524, -57.5809) -> (61.4337, -57.5912) projected
  line L352 (61.4337, -57.5912) -> (61.5163, -57.5974) projected
  line L353 (61.5163, -57.5974) -> (61.5999, -57.5995) projected
  line L354 (61.5999, -57.5995) -> (61.6835, -57.5974) projected
  line L355 (61.6835, -57.5974) -> (61.766, -57.5911) projected
  line L356 (61.766, -57.5911) -> (61.8474, -57.5807) projected
  line L357 (61.8474, -57.5807) -> (61.9274, -57.5664) projected
  line L358 (61.9274, -57.5664) -> (62.006, -57.5482) projected
  line L359 (62.006, -57.5482) -> (62.0831, -57.5263) projected
  line L360 (62.0831, -57.5263) -> (62.1586, -57.5008) projected
  line L361 (62.1586, -57.5008) -> (62.2324, -57.4716) projected
  line L362 (62.2324, -57.4716) -> (62.3044, -57.4391) projected
  line L363 (62.3044, -57.4391) -> (62.3744, -57.4032) projected
  line L364 (62.3744, -57.4032) -> (62.4424, -57.364) projected
  line L365 (62.4424, -57.364) -> (62.5084, -57.3217) projected
  line L366 (62.5084, -57.3217) -> (62.5721, -57.2764) projected
  line L367 (62.5721, -57.2764) -> (62.6334, -57.2282) projected
  line L368 (62.6334, -57.2282) -> (62.6924, -57.1771) projected
  line L369 (62.6924, -57.1771) -> (62.7488, -57.1232) projected
  line L370 (62.7488, -57.1232) -> (62.8026, -57.0668) projected
  line L371 (62.8026, -57.0668) -> (62.8537, -57.0078) projected
  line L372 (62.8537, -57.0078) -> (62.9019, -56.9464) projected
  line L373 (62.9019, -56.9464) -> (62.9472, -56.8827) projected
  line L374 (62.9472, -56.8827) -> (62.9894, -56.8167) projected
  line L375 (62.9894, -56.8167) -> (63.0285, -56.7487) projected
  line L376 (63.0285, -56.7487) -> (63.0644, -56.6786) projected
  line L377 (63.0644, -56.6786) -> (63.0969, -56.6066) projected
  line L378 (63.0969, -56.6066) -> (63.126, -56.5328) projected
  line L379 (63.126, -56.5328) -> (63.1515, -56.4573) projected
  line L380 (63.1515, -56.4573) -> (63.1734, -56.3802) projected
  line L381 (63.1734, -56.3802) -> (63.1915, -56.3016) projected
  line L382 (63.1915, -56.3016) -> (63.2058, -56.2215) projected
  line L383 (63.2058, -56.2215) -> (63.2161, -56.1402) projected
  line L384 (67.06, -63.215) -> (67.1425, -63.2212) projected
  line L385 (67.1425, -63.2212) -> (67.2261, -63.2233) projected
  line L386 (67.2261, -63.2233) -> (67.3097, -63.2211) projected
  line L387 (67.3097, -63.2211) -> (67.3923, -63.2148) projected
  line L388 (67.3923, -63.2148) -> (67.4736, -63.2045) projected
  line L389 (67.4736, -63.2045) -> (67.5536, -63.1902) projected
  line L390 (67.5536, -63.1902) -> (67.6322, -63.172) projected
  line L391 (67.6322, -63.172) -> (67.7093, -63.15) projected
  line L392 (67.7093, -63.15) -> (67.7848, -63.1245) projected
  line L393 (67.7848, -63.1245) -> (67.8586, -63.0953) projected
  line L394 (67.8586, -63.0953) -> (67.9306, -63.0628) projected
  line L395 (67.9306, -63.0628) -> (68.0006, -63.0269) projected
  line L396 (68.0006, -63.0269) -> (68.0686, -62.9877) projected
  line L397 (68.0686, -62.9877) -> (68.1346, -62.9454) projected
  line L398 (68.1346, -62.9454) -> (68.1982, -62.9001) projected
  line L399 (68.1982, -62.9001) -> (68.2596, -62.8518) projected
  line L400 (68.2596, -62.8518) -> (68.3186, -62.8007) projected
  line L401 (68.3186, -62.8007) -> (68.375, -62.7469) projected
  line L402 (68.375, -62.7469) -> (68.4288, -62.6904) projected
  line L403 (68.4288, -62.6904) -> (68.4798, -62.6314) projected
  line L404 (68.4798, -62.6314) -> (68.528, -62.57) projected
  line L405 (68.528, -62.57) -> (68.5733, -62.5063) projected
  line L406 (68.5733, -62.5063) -> (68.6155, -62.4404) projected
  line L407 (68.6155, -62.4404) -> (68.6546, -62.3723) projected
  line L408 (68.6546, -62.3723) -> (68.6905, -62.3022) projected
  line L409 (68.6905, -62.3022) -> (68.723, -62.2302) projected
  line L410 (68.723, -62.2302) -> (68.7521, -62.1564) projected
  line L411 (68.7521, -62.1564) -> (68.7776, -62.0809) projected
  line L412 (68.7776, -62.0809) -> (68.7995, -62.0038) projected
  line L413 (68.7995, -62.0038) -> (68.8176, -61.9252) projected
  line L414 (68.8176, -61.9252) -> (68.8318, -61.8451) projected
  line L415 (68.8318, -61.8451) -> (68.8421, -61.7638) projected
  line L416 (68.8421, -61.7638) -> (68.8484, -61.6813) projected
  line L417 (68.8484, -61.6813) -> (68.8505, -61.5976) projected
  line L418 (68.8505, -61.5976) -> (68.8483, -61.514) projected
  line L419 (68.8483, -61.514) -> (68.842, -61.4315) projected
  line L420 (68.842, -61.4315) -> (68.8316, -61.3502) projected
  line L421 (68.8316, -61.3502) -> (68.8173, -61.2702) projected
  line L422 (68.8173, -61.2702) -> (68.7991, -61.1916) projected
  line L423 (68.7991, -61.1916) -> (68.7772, -61.1144) projected
  line L424 (68.7772, -61.1144) -> (68.7516, -61.039) projected
  line L425 (68.7516, -61.039) -> (68.7225, -60.9652) projected
  line L426 (68.7225, -60.9652) -> (68.6899, -60.8932) projected
  line L427 (68.6899, -60.8932) -> (68.654, -60.8232) projected
  line L428 (68.654, -60.8232) -> (68.6149, -60.7551) projected
  line L429 (68.6149, -60.7551) -> (68.5726, -60.6892) projected
  line L430 (68.5726, -60.6892) -> (68.5272, -60.6255) projected
  line L431 (68.5272, -60.6255) -> (68.479, -60.5641) projected
  line L432 (68.479, -60.5641) -> (68.4279, -60.5052) projected
  line L433 (68.4279, -60.5052) -> (68.374, -60.4488) projected
  line L434 (68.374, -60.4488) -> (68.3176, -60.395) projected
  line L435 (68.3176, -60.395) -> (68.2586, -60.344) projected
  line L436 (68.2586, -60.344) -> (68.1972, -60.2957) projected
  line L437 (68.1972, -60.2957) -> (68.1335, -60.2505) projected
  line L438 (68.1335, -60.2505) -> (68.0675, -60.2082) projected
  line L439 (68.0675, -60.2082) -> (67.9995, -60.1691) projected
  line L440 (67.9995, -60.1691) -> (67.9294, -60.1333) projected
  line L441 (67.9294, -60.1333) -> (67.8574, -60.1007) projected
  line L442 (67.8574, -60.1007) -> (67.7836, -60.0717) projected
  line L443 (67.7836, -60.0717) -> (67.7081, -60.0462) projected
  line L444 (67.7081, -60.0462) -> (67.6309, -60.0243) projected
  line L445 (67.6309, -60.0243) -> (67.5523, -60.0062) projected
  line L446 (67.5523, -60.0062) -> (67.4723, -59.9919) projected
  line L447 (67.4723, -59.9919) -> (67.391, -59.9816) projected
  line L448 (67.391, -59.9816) -> (67.3084, -59.9754) projected
  line L449 (67.3084, -59.9754) -> (67.2248, -59.9733) projected
  line L450 (67.2248, -59.9733) -> (67.1412, -59.9754) projected
  line L451 (67.1412, -59.9754) -> (67.0587, -59.9818) projected
  line L452 (67.0587, -59.9818) -> (66.9773, -59.9921) projected
  line L453 (66.9773, -59.9921) -> (66.8973, -60.0064) projected
  line L454 (66.8973, -60.0064) -> (66.8187, -60.0246) projected
  line L455 (66.8187, -60.0246) -> (66.7416, -60.0465) projected
  line L456 (66.7416, -60.0465) -> (66.6661, -60.0721) projected
  line L457 (66.6661, -60.0721) -> (66.5923, -60.1013) projected
  line L458 (66.5923, -60.1013) -> (66.5204, -60.1338) projected
  line L459 (66.5204, -60.1338) -> (66.4503, -60.1697) projected
  line L460 (66.4503, -60.1697) -> (66.3823, -60.2089) projected
  line L461 (66.3823, -60.2089) -> (66.3164, -60.2512) projected
  line L462 (66.3164, -60.2512) -> (66.2527, -60.2965) projected
  line L463 (66.2527, -60.2965) -> (66.1913, -60.3448) projected
  line L464 (66.1913, -60.3448) -> (66.1324, -60.3959) projected
  line L465 (66.1324, -60.3959) -> (66.0759, -60.4497) projected
  line L466 (66.0759, -60.4497) -> (66.0222, -60.5062) projected
  line L467 (66.0222, -60.5062) -> (65.9711, -60.5652) projected
  line L468 (65.9711, -60.5652) -> (65.9229, -60.6266) projected
  line L469 (65.9229, -60.6266) -> (65.8776, -60.6903) projected
  line L470 (65.8776, -60.6903) -> (65.8354, -60.7562) projected
  line L471 (65.8354, -60.7562) -> (65.7963, -60.8243) projected
  line L472 (65.7963, -60.8243) -> (65.7604, -60.8944) projected
  line L473 (65.7604, -60.8944) -> (65.7279, -60.9664) projected
  line L474 (65.7279, -60.9664) -> (65.6988, -61.0402) projected
  line L475 (65.6988, -61.0402) -> (65.6733, -61.1157) projected
  line L476 (65.6733, -61.1157) -> (65.6515, -61.1928) projected
  line L477 (65.6515, -61.1928) -> (65.6333, -61.2714) projected
  line L478 (65.6333, -61.2714) -> (65.6191, -61.3515) projected
  line L479 (65.6191, -61.3515) -> (65.6088, -61.4328) projected
  line L480 (65.6088, -61.4328) -> (65.6025, -61.5153) projected
  line L481 (65.6025, -61.5153) -> (65.6005, -61.599) projected
  line L482 (65.6005, -61.599) -> (65.6026, -61.6826) projected
  line L483 (65.6026, -61.6826) -> (65.6089, -61.7651) projected
  line L484 (65.6089, -61.7651) -> (65.6193, -61.8464) projected
  line L485 (65.6193, -61.8464) -> (65.6336, -61.9264) projected
  line L486 (65.6336, -61.9264) -> (65.6518, -62.005) projected
  line L487 (65.6518, -62.005) -> (65.6737, -62.0821) projected
  line L488 (65.6737, -62.0821) -> (65.6993, -62.1576) projected
  line L489 (65.6993, -62.1576) -> (65.7284, -62.2314) projected
  line L490 (65.7284, -62.2314) -> (65.761, -62.3034) projected
  line L491 (65.761, -62.3034) -> (65.7969, -62.3734) projected
  line L492 (65.7969, -62.3734) -> (65.8361, -62.4415) projected
  line L493 (65.8361, -62.4415) -> (65.8783, -62.5074) projected
  line L494 (65.8783, -62.5074) -> (65.9237, -62.5711) projected
  line L495 (65.9237, -62.5711) -> (65.9719, -62.6325) projected
  line L496 (65.9719, -62.6325) -> (66.023, -62.6914) projected
  line L497 (66.023, -62.6914) -> (66.0769, -62.7478) projected
  line L498 (66.0769, -62.7478) -> (66.1333, -62.8016) projected
  line L499 (66.1333, -62.8016) -> (66.1923, -62.8526) projected
  line L500 (66.1923, -62.8526) -> (66.2537, -62.9009) projected
  line L501 (66.2537, -62.9009) -> (66.3174, -62.9461) projected
  line L502 (66.3174, -62.9461) -> (66.3834, -62.9884) projected
  line L503 (66.3834, -62.9884) -> (66.4515, -63.0275) projected
  line L504 (66.4515, -63.0275) -> (66.5215, -63.0633) projected
  line L505 (66.5215, -63.0633) -> (66.5935, -63.0959) projected
  line L506 (66.5935, -63.0959) -> (66.6673, -63.1249) projected
  line L507 (66.6673, -63.1249) -> (66.7429, -63.1504) projected
  line L508 (66.7429, -63.1504) -> (66.82, -63.1723) projected
  line L509 (66.82, -63.1723) -> (66.8986, -63.1904) projected
  line L510 (66.8986, -63.1904) -> (66.9786, -63.2047) projected
  line L511 (66.9786, -63.2047) -> (67.06, -63.215) projected
  line L512 (59.9853, -67.0602) -> (59.9791, -67.1428) projected
  line L513 (59.9791, -67.1428) -> (59.977, -67.2264) projected
  line L514 (59.977, -67.2264) -> (59.9792, -67.31) projected
  line L515 (59.9792, -67.31) -> (59.9855, -67.3925) projected
  line L516 (59.9855, -67.3925) -> (59.9958, -67.4738) projected
  line L517 (59.9958, -67.4738) -> (60.0102, -67.5539) projected
  line L518 (60.0102, -67.5539) -> (60.0284, -67.6325) projected
  line L519 (60.0284, -67.6325) -> (60.0503, -67.7096) projected
  line L520 (60.0503, -67.7096) -> (60.0759, -67.7851) projected
  line L521 (60.0759, -67.7851) -> (60.105, -67.8588) projected
  line L522 (60.105, -67.8588) -> (60.1376, -67.9308) projected
  line L523 (60.1376, -67.9308) -> (60.1735, -68.0009) projected
  line L524 (60.1735, -68.0009) -> (60.2126, -68.0689) projected
  line L525 (60.2126, -68.0689) -> (60.2549, -68.1348) projected
  line L526 (60.2549, -68.1348) -> (60.3003, -68.1985) projected
  line L527 (60.3003, -68.1985) -> (60.3486, -68.2599) projected
  line L528 (60.3486, -68.2599) -> (60.3997, -68.3188) projected
  line L529 (60.3997, -68.3188) -> (60.4535, -68.3752) projected
  line L530 (60.4535, -68.3752) -> (60.5099, -68.429) projected
  line L531 (60.5099, -68.429) -> (60.5689, -68.48) projected
  line L532 (60.5689, -68.48) -> (60.6303, -68.5283) projected
  line L533 (60.6303, -68.5283) -> (60.6941, -68.5735) projected
  line L534 (60.6941, -68.5735) -> (60.76, -68.6158) projected
  line L535 (60.76, -68.6158) -> (60.8281, -68.6549) projected
  line L536 (60.8281, -68.6549) -> (60.8982, -68.6907) projected
  line L537 (60.8982, -68.6907) -> (60.9702, -68.7232) projected
  line L538 (60.9702, -68.7232) -> (61.044, -68.7523) projected
  line L539 (61.044, -68.7523) -> (61.1195, -68.7778) projected
  line L540 (61.1195, -68.7778) -> (61.1966, -68.7997) projected
  line L541 (61.1966, -68.7997) -> (61.2752, -68.8178) projected
  line L542 (61.2752, -68.8178) -> (61.3553, -68.832) projected
  line L543 (61.3553, -68.832) -> (61.4366, -68.8423) projected
  line L544 (61.4366, -68.8423) -> (61.5191, -68.8486) projected
  line L545 (61.5191, -68.8486) -> (61.6028, -68.8506) projected
  line L546 (61.6028, -68.8506) -> (61.6864, -68.8485) projected
  line L547 (61.6864, -68.8485) -> (61.7689, -68.8422) projected
  line L548 (61.7689, -68.8422) -> (61.8502, -68.8318) projected
  line L549 (61.8502, -68.8318) -> (61.9302, -68.8175) projected
  line L550 (61.9302, -68.8175) -> (62.0088, -68.7993) projected
  line L551 (62.0088, -68.7993) -> (62.0859, -68.7774) projected
  line L552 (62.0859, -68.7774) -> (62.1614, -68.7518) projected
  line L553 (62.1614, -68.7518) -> (62.2352, -68.7226) projected
  line L554 (62.2352, -68.7226) -> (62.3072, -68.6901) projected
  line L555 (62.3072, -68.6901) -> (62.3772, -68.6542) projected
  line L556 (62.3772, -68.6542) -> (62.4453, -68.615) projected
  line L557 (62.4453, -68.615) -> (62.5112, -68.5727) projected
  line L558 (62.5112, -68.5727) -> (62.5749, -68.5274) projected
  line L559 (62.5749, -68.5274) -> (62.6362, -68.4791) projected
  line L560 (62.6362, -68.4791) -> (62.6952, -68.428) projected
  line L561 (62.6952, -68.428) -> (62.7516, -68.3742) projected
  line L562 (62.7516, -68.3742) -> (62.8054, -68.3177) projected
  line L563 (62.8054, -68.3177) -> (62.8564, -68.2587) projected
  line L564 (62.8564, -68.2587) -> (62.9046, -68.1973) projected
  line L565 (62.9046, -68.1973) -> (62.9499, -68.1336) projected
  line L566 (62.9499, -68.1336) -> (62.9921, -68.0676) projected
  line L567 (62.9921, -68.0676) -> (63.0312, -67.9996) projected
  line L568 (63.0312, -67.9996) -> (63.0671, -67.9295) projected
  line L569 (63.0671, -67.9295) -> (63.0996, -67.8575) projected
  line L570 (63.0996, -67.8575) -> (63.1287, -67.7837) projected
  line L571 (63.1287, -67.7837) -> (63.1542, -67.7082) projected
  line L572 (63.1542, -67.7082) -> (63.176, -67.631) projected
  line L573 (63.176, -67.631) -> (63.1941, -67.5524) projected
  line L574 (63.1941, -67.5524) -> (63.2084, -67.4724) projected
  line L575 (63.2084, -67.4724) -> (63.2187, -67.391) projected
  line L576 (63.2187, -67.391) -> (63.2249, -67.3085) projected
  line L577 (63.2249, -67.3085) -> (63.227, -67.2249) projected
  line L578 (63.227, -67.2249) -> (63.2249, -67.1413) projected
  line L579 (63.2249, -67.1413) -> (63.2185, -67.0588) projected
  line L580 (63.2185, -67.0588) -> (63.2082, -66.9774) projected
  line L581 (63.2082, -66.9774) -> (63.1938, -66.8974) projected
  line L582 (63.1938, -66.8974) -> (63.1757, -66.8188) projected
  line L583 (63.1757, -66.8188) -> (63.1537, -66.7417) projected
  line L584 (63.1537, -66.7417) -> (63.1281, -66.6662) projected
  line L585 (63.1281, -66.6662) -> (63.099, -66.5924) projected
  line L586 (63.099, -66.5924) -> (63.0664, -66.5205) projected
  line L587 (63.0664, -66.5205) -> (63.0305, -66.4504) projected
  line L588 (63.0305, -66.4504) -> (62.9914, -66.3824) projected
  line L589 (62.9914, -66.3824) -> (62.9491, -66.3165) projected
  line L590 (62.9491, -66.3165) -> (62.9037, -66.2528) projected
  line L591 (62.9037, -66.2528) -> (62.8555, -66.1914) projected
  line L592 (62.8555, -66.1914) -> (62.8044, -66.1325) projected
  line L593 (62.8044, -66.1325) -> (62.7505, -66.0761) projected
  line L594 (62.7505, -66.0761) -> (62.6941, -66.0223) projected
  line L595 (62.6941, -66.0223) -> (62.6351, -65.9712) projected
  line L596 (62.6351, -65.9712) -> (62.5737, -65.923) projected
  line L597 (62.5737, -65.923) -> (62.5099, -65.8777) projected
  line L598 (62.5099, -65.8777) -> (62.444, -65.8355) projected
  line L599 (62.444, -65.8355) -> (62.3759, -65.7964) projected
  line L600 (62.3759, -65.7964) -> (62.3058, -65.7606) projected
  line L601 (62.3058, -65.7606) -> (62.2338, -65.7281) projected
  line L602 (62.2338, -65.7281) -> (62.16, -65.699) projected
  line L603 (62.16, -65.699) -> (62.0845, -65.6735) projected
  line L604 (62.0845, -65.6735) -> (62.0074, -65.6516) projected
  line L605 (62.0074, -65.6516) -> (61.9288, -65.6335) projected
  line L606 (61.9288, -65.6335) -> (61.8487, -65.6193) projected
  line L607 (61.8487, -65.6193) -> (61.7674, -65.609) projected
  line L608 (61.7674, -65.609) -> (61.6849, -65.6027) projected
  line L609 (61.6849, -65.6027) -> (61.6013, -65.6006) projected
  line L610 (61.6013, -65.6006) -> (61.5176, -65.6028) projected
  line L611 (61.5176, -65.6028) -> (61.4351, -65.6091) projected
  line L612 (61.4351, -65.6091) -> (61.3538, -65.6195) projected
  line L613 (61.3538, -65.6195) -> (61.2738, -65.6338) projected
  line L614 (61.2738, -65.6338) -> (61.1952, -65.652) projected
  line L615 (61.1952, -65.652) -> (61.1181, -65.6739) projected